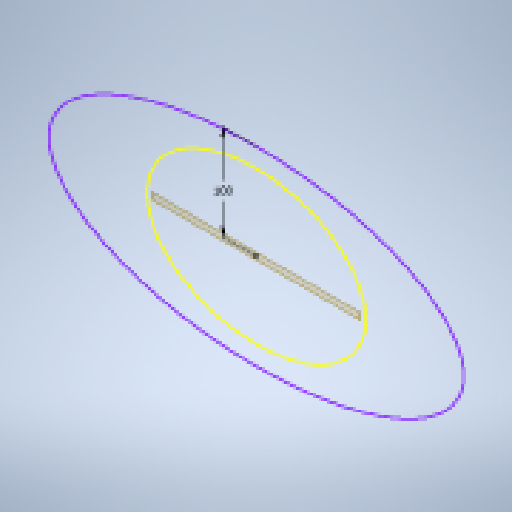
# Autodesk Inventor part: Верхний эллипс
Saved by Autodesk Inventor 2023.1 (Build 271208000, 208)
## iProperties
Created: 2024-11-20
Part Number: Верхний эллипс
Material: Типовые
Document SubType Name: Modeling
Designer: DELL
Density: 1 g/cm^3
Appearance: По умолчанию
Author: DELL
Autodesk Inventor part; units mm, degrees
ref_plane "YZ Plane" through (0, 0, 0) normal (1, 0, 0) x (0, 1, 0)
ref_plane "XZ Plane" through (0, 0, 0) normal (0, 1, 0) x (-1, 0, 0)
ref_plane "XY Plane" through (0, 0, 0) normal (0, 0, 1) x (1, 0, 0)
ref_plane "РабПлоскость1" through (0, 0, 0) normal (0, 0, 1) x (1, 0, 0)
sketch "Эскиз1" plane through (0, 0, 0) normal (0, 0, 1) x (1, 0, 0)
  ellipse E0 centre (0, 0) end of major axis (-119.9976, 0.7623) minor radius 79.9991 construction
  ellipse E1 centre (0, 0) end of major axis (100, 0) minor radius 70
  point P0 (0, 0)
  point P1 (100, 0)
  dimension "d0" = 70
  dimension "d1" = 100
  constraints: 1 coincident, 1 horizontal alignment, 3 other
  measures "d1" distance of point (100, 0) point (0, 0)
extrude "Выдавливание1" add sketch "Эскиз1" against normal blind 4
